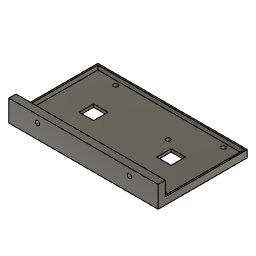
Support supérieur arduino v4 (Autodesk Fusion 360 design; units mm, degrees)
Autodesk Fusion 360 part; units mm, degrees
sketch "Esquisse2" plane through (0, 0, 0) normal (0, 0, 1) x (1, 0, 0)
  line L0 (0, 0) -> (104, 0)
  line L1 (104, 0) -> (104, 56)
  line L2 (104, 56) -> (0, 56)
  line L3 (0, 56) -> (0, 0)
  dimension "d1" = 104
  dimension "d2" = 56
  constraint horizontal L0
  constraint vertical L1
  constraint horizontal L2
  constraint vertical L3
  constraint coincident L0.start L3.end
  measures "d1" distance of L1.end L2.end
  measures "d2" distance of L0.end L1.end
extrude "Extrusion1" add sketch "Esquisse2" along normal blind 2
sketch "Esquisse3" plane through (0, 0, 2) normal (0, 0, 1) x (-1, 0, 0)
  line L0 (0, -56) -> (0, 0)
  line L1 (0, 0) -> (-104, 0)
  line L2 (-104, 0) -> (-104, -56)
  line L3 (-104, -56) -> (0, -56)
  line L4 (0, -56) -> (-104, -56)
  line L5 (-104, -56) -> (-104, 0)
  line L6 (-104, 0) -> (0, 0)
  line L7 (0, 0) -> (0, -56)
  line L8 (-1, -55) -> (-103, -55)
  line L9 (-103, -55) -> (-103, -1)
  line L10 (-103, -1) -> (-1, -1)
  line L11 (-1, -1) -> (-1, -55)
  dimension "d5" = 1
  dimension "d6" = 1
  dimension "d7" = 1
  dimension "d8" = 1
  constraint horizontal L4
  constraint vertical L5
  constraint horizontal L6
  constraint vertical L7
  constraint coincident L1.end L2.start
  constraint coincident L0.start L3.end
  constraint horizontal L8
  constraint vertical L9
  constraint horizontal L10
  constraint vertical L11
  measures "d5" distance of L4 L8
  measures "d6" distance of L7 L11
  measures "d7" distance of L6 L10
  measures "d8" distance of L5 L9
extrude "Extrusion2" add sketch "Esquisse3" along normal blind 3
sketch "Esquisse4" plane through (0, 0, 2) normal (0, 0, 1) x (-1, 0, 0)
  line L0 (-103, -1) -> (-103, -55)
  line L1 (-103, -55) -> (-1, -55)
  line L2 (-1, -55) -> (-1, -1)
  line L3 (-1, -1) -> (-103, -1)
  circle A0 centre (-16.5, -52) radius 1.5
  circle A1 centre (-15.5, -4) radius 1.5
  circle A2 centre (-67.5, -37.5) radius 1.5
  circle A3 centre (-67.5, -9) radius 1.5
  circle A4 centre (-91.5, -52) radius 1.5
  circle A5 centre (-97.5, -4) radius 1.5
  dimension "d11" = 3
  dimension "d12" = 3
  dimension "d13" = 3
  dimension "d14" = 3
  dimension "d15" = 3
  dimension "d16" = 3
  dimension "d17" = 3
  dimension "d18" = 15.5
  dimension "d19" = 3
  dimension "d20" = 14.5
  dimension "d21" = 35.5
  dimension "d22" = 17.5
  dimension "d23" = 35.5
  dimension "d24" = 8
  dimension "d25" = 11.5
  dimension "d26" = 3
  dimension "d27" = 3
  dimension "d28" = 5.5
  measures "d11" distance of L1 A0.centre
  measures "d12" diameter of A0
  measures "d13" diameter of A4
  measures "d14" diameter of A2
  measures "d15" diameter of A3
  measures "d16" diameter of A5
  measures "d17" diameter of A1
  measures "d18" distance of L2 A0.centre
  measures "d19" distance of L3 A1.centre
  measures "d20" distance of L2 A1.centre
  measures "d21" distance of L0 A2.centre
  measures "d22" distance of L1 A2.centre
  measures "d23" distance of L0 A3.centre
  measures "d24" distance of L3 A3.centre
  measures "d25" distance of L0 A4.centre
  measures "d26" distance of L1 A4.centre
  measures "d27" distance of L3 A5.centre
  measures "d28" distance of L0 A5.centre
extrude "Extrusion3" cut sketch "Esquisse4" against normal blind 5 contours A0 | A1 | A2 | A3 | A4 | A5
sketch "Esquisse6" plane through (0, 0, 0) normal (0, 0, -1) x (1, 0, 0)
  circle A0 centre (15.5, -4) radius 1.5
  circle A1 centre (91.5, -52) radius 1.5
  circle A2 centre (67.5, -9) radius 1.5
  circle A3 centre (16.5, -52) radius 1.5
  circle A4 centre (67.5, -37.5) radius 1.5
  circle A5 centre (97.5, -4) radius 1.5
  line L0 (0, 0) -> (0, -56)
  line L1 (0, -56) -> (104, -56)
  line L2 (104, -56) -> (104, 0)
  line L3 (104, 0) -> (0, 0)
  line L4 (20, -23) -> (30, -23)
  line L5 (30, -23) -> (30, -33)
  line L6 (30, -33) -> (20, -33)
  line L7 (20, -33) -> (20, -23)
  line L8 (74, -23) -> (84, -23)
  line L9 (84, -23) -> (84, -33)
  line L10 (84, -33) -> (74, -33)
  line L11 (74, -33) -> (74, -23)
  dimension "d34" = 10
  dimension "d35" = 10
  dimension "d36" = 10
  dimension "d37" = 10
  dimension "d38" = 20
  dimension "d39" = 23
  dimension "d40" = 23
  dimension "d41" = 20
  constraint horizontal L4
  constraint vertical L5
  constraint horizontal L6
  constraint vertical L7
  constraint horizontal L8
  constraint vertical L9
  constraint horizontal L10
  constraint vertical L11
  measures "d34" distance of L4.start L4.end
  measures "d35" distance of L4.end L5.end
  measures "d36" distance of L8.start L8.end
  measures "d37" distance of L8.end L9.end
  measures "d38" distance of L2 L9
  measures "d39" distance of L3 L8
  measures "d40" distance of L3 L4
  measures "d41" distance of L0 L7
extrude "Extrusion4" cut sketch "Esquisse6" against normal blind 5 contours L4 L5 L6 L7 | L8 L9 L10 L11
sketch "Esquisse7" plane through (0, 0, 0) normal (0, -1, 0) x (1, 0, 0)
  line L0 (0, 0) -> (104, 0)
  line L1 (104, 0) -> (104, 5)
  line L2 (104, 5) -> (0, 5)
  line L3 (0, 5) -> (0, 0)
  line L4 (0, 0) -> (104, 0)
  line L5 (104, 0) -> (104, 5)
  line L6 (104, 5) -> (0, 5)
  line L7 (0, 5) -> (0, 0)
  constraint horizontal L4
  constraint vertical L5
  constraint horizontal L6
  constraint vertical L7
  constraint coincident L1.end L2.start
  constraint coincident L0.start L3.end
extrude "Extrusion5" add sketch "Esquisse7" along normal blind 6
sketch "Esquisse8" plane through (0, 0, 5) normal (0, 0, 1) x (-1, 0, 0)
  line L0 (-103, -1) -> (-1, -1)
  line L1 (-1, -1) -> (-1, -55)
  line L2 (-1, -55) -> (-103, -55)
  line L3 (-103, -55) -> (-103, -1)
  line L4 (-104, 6) -> (-104, -56)
  line L5 (-104, -56) -> (0, -56)
  line L6 (0, -56) -> (0, 6)
  line L7 (0, 6) -> (-104, 6)
  line L8 (0, 6) -> (-104, 6)
  line L9 (-104, 6) -> (-104, 1)
  line L10 (-104, 1) -> (0, 1)
  line L11 (0, 1) -> (0, 6)
  dimension "d46" = 5
  constraint horizontal L8
  constraint vertical L9
  constraint horizontal L10
  constraint vertical L11
  constraint coincident L4 L9.end
  constraint coincident L6.end L7.start
  measures "d46" distance of L4.start L9.end
extrude "Extrusion6" add sketch "Esquisse8" along normal blind 10 contours L4 L6 L7 L8 L9 L10 L11
sketch "Esquisse9" plane through (0, -1, 0) normal (0, 1, 0) x (-1, 0, 0)
  line L0 (-104, 5) -> (0, 5)
  line L1 (0, 5) -> (0, 15)
  line L2 (0, 15) -> (-104, 15)
  line L3 (-104, 15) -> (-104, 5)
  circle A0 centre (-20, 10) radius 1.5
  circle A1 centre (-84, 10) radius 1.5
  dimension "d49" = 3
  dimension "d50" = 3
  dimension "d51" = 20
  dimension "d52" = 20
  dimension "d53" = 5
  dimension "d54" = 5
  measures "d49" diameter of A1
  measures "d50" diameter of A0
  measures "d51" distance of L3 A1.centre
  measures "d52" distance of L1 A0.centre
  measures "d53" distance of L2 A1.centre
  measures "d54" distance of L2 A0.centre
extrude "Extrusion7" cut sketch "Esquisse9" against normal blind 5 contours A0 | A1
